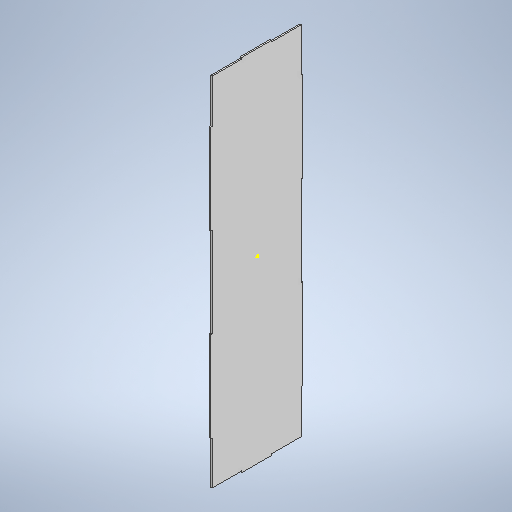
# Autodesk Inventor part: PAREDES LATERAIS
Saved by Autodesk Inventor 2025.2 (Build 292293000, 293)
## iProperties
Created: 2025-05-08
Part Number: PAREDES LATERAIS
Material: Genérico
Document SubType Name: Modeling
Designer: erick
Density: 1 g/cm^3
Appearance: Padrão
Author: erick
Autodesk Inventor part; units mm, degrees
ref_plane "YZ Plane" through (0, 0, 0) normal (1, 0, 0) x (0, 1, 0)
ref_plane "XZ Plane" through (0, 0, 0) normal (0, 1, 0) x (-1, 0, 0)
ref_plane "XY Plane" through (0, 0, 0) normal (0, 0, 1) x (1, 0, 0)
sketch "Esboço1" plane through (0, 0, 0) normal (1, 0, 0) x (0, 1, 0)
  line L0 (-504, 129) -> (504, 129)
  line L1 (504, 129) -> (504, -129)
  line L2 (504, -129) -> (-504, -129)
  line L3 (-504, -129) -> (-504, 129)
  line L4 (-504, 129) -> (504, -129) construction
  line L5 (504, 129) -> (-504, -129) construction
  point P0 (0, 0)
  dimension "d0" = 1008
  dimension "d1" = 258
  constraints: 12 end point, 2 midpoint, 2 parallel, 1 horizontal, 1 perpendicular
  measures "d0" distance of L1.end L2.end
  measures "d1" distance of L0.end L1.end
extrude "Extrusão1" add sketch "Esboço1" along normal mid plane 4
sketch "Esboço3" plane through (2, 0, 0) normal (1, 0, 0) x (0, 0, -1)
  line L0 (-133, 630) -> (-125, 630)
  line L1 (-125, 630) -> (-125, 378)
  line L2 (-125, 378) -> (-133, 378)
  line L3 (-133, 378) -> (-133, 630)
  line L4 (129, 504) -> (-129, 504) projected
  line L5 (-133, 630) -> (-125, 378) construction
  line L6 (-125, 630) -> (-133, 378) construction
  line L7 (-125, 126) -> (-133, 126)
  line L8 (-133, 126) -> (-133, -126)
  line L9 (-133, -126) -> (-125, -126)
  line L10 (-125, -126) -> (-125, 126)
  line L11 (-129, 504) -> (-129, -504) projected
  line L12 (-125, 126) -> (-133, -126) construction
  line L13 (-133, 126) -> (-125, -126) construction
  line L14 (-125, -378) -> (-133, -378)
  line L15 (-133, -378) -> (-133, -630)
  line L16 (-133, -630) -> (-125, -630)
  line L17 (-125, -630) -> (-125, -378)
  line L18 (-125, -378) -> (-133, -630) construction
  line L19 (-133, -378) -> (-125, -630) construction
  line L20 (125, 630) -> (133, 630)
  line L21 (133, 630) -> (133, 378)
  line L22 (133, 378) -> (125, 378)
  line L23 (125, 378) -> (125, 630)
  line L24 (125, 630) -> (133, 378) construction
  line L25 (133, 630) -> (125, 378) construction
  line L26 (125, 126) -> (133, 126)
  line L27 (133, 126) -> (133, -126)
  line L28 (133, -126) -> (125, -126)
  line L29 (125, -126) -> (125, 126)
  line L30 (129, -504) -> (129, 504) projected
  line L31 (125, 126) -> (133, -126) construction
  line L32 (133, 126) -> (125, -126) construction
  line L33 (125, -378) -> (133, -378)
  line L34 (133, -378) -> (133, -630)
  line L35 (133, -630) -> (125, -630)
  line L36 (125, -630) -> (125, -378)
  line L37 (125, -378) -> (133, -630) construction
  line L38 (133, -378) -> (125, -630) construction
  point P0 (0, 0)
  point P1 (-129, 0)
  point P2 (-129, -504)
  point P3 (129, 0)
  dimension "d8" = 8
  dimension "d9" = 252
  dimension "d10" = 252
  dimension "d11" = 252
  dimension "d12" = 8
  dimension "d13" = 252
  dimension "d14" = 8
  dimension "d15" = 252
  dimension "d16" = 8
  dimension "d17" = 252
  dimension "d18" = 252
  dimension "d19" = 8
  dimension "d20" = 252
  dimension "d21" = 252
  dimension "d22" = 8
  dimension "d23" = 252
  constraints: 72 end point, 14 midpoint, 12 parallel, 6 horizontal, 6 perpendicular, 1 point on line
  measures "d8" distance of L0.start L0.end
  measures "d9" distance of L0.end L1.end
  measures "d10" distance of L9.end L7.start
  measures "d11" distance between parallel lines of L7 L2
  measures "d12" distance of L8.end L9.end
  measures "d13" distance between parallel lines of L14 L9
  measures "d14" distance of L14.start L14.end
  measures "d15" distance of L16.end L14.start
  measures "d16" distance of L21.end L22.end
  measures "d17" distance of L20.end L21.end
  measures "d18" distance between parallel lines of L26 L22
  measures "d19" distance of L26.start L26.end
  measures "d20" distance of L26.end L27.end
  measures "d21" distance of L33.end L34.end
  measures "d22" distance of L33.start L33.end
  measures "d23" distance between parallel lines of L33 L28
extrude "Extrusão3" cut sketch "Esboço3" along normal through all both and the other way through all
sketch "Esboço4" plane through (2, 0, 0) normal (1, 0, 0) x (0, 0, -1)
  line L0 (-125, 504) -> (125, 504) projected
  line L1 (-125, 504) -> (-42, 504)
  line L2 (-42, 504) -> (-42, 500)
  line L3 (-42, 500) -> (-125, 500)
  line L4 (-125, 500) -> (-125, 504)
  line L5 (125, 504) -> (42, 504)
  line L6 (42, 504) -> (42, 500)
  line L7 (42, 500) -> (125, 500)
  line L8 (125, 500) -> (125, 504)
  line L9 (-125, -504) -> (125, -504) projected
  line L10 (-125, -504) -> (-42, -504)
  line L11 (-42, -504) -> (-42, -500)
  line L12 (-42, -500) -> (-125, -500)
  line L13 (-125, -500) -> (-125, -504)
  line L14 (125, -504) -> (42, -504)
  line L15 (42, -504) -> (42, -500)
  line L16 (42, -500) -> (125, -500)
  line L17 (125, -500) -> (125, -504)
  point P0 (0, 0)
  dimension "d26" = 83
  dimension "d27" = 4
  dimension "d28" = 83
  dimension "d29" = 4
  dimension "d30" = 84
  dimension "d31" = 83
  dimension "d32" = 4
  dimension "d33" = 83
  dimension "d34" = 4
  dimension "d35" = 84
  constraints: 32 end point, 8 parallel, 4 horizontal, 4 perpendicular
  measures "d26" distance of L2.end L3.end
  measures "d27" distance of L1.end L2.end
  measures "d28" distance of L6.end L7.end
  measures "d29" distance of L5.end L6.end
  measures "d30" distance between parallel lines of L6 L2
  measures "d31" distance of L11.end L12.end
  measures "d32" distance of L10.end L11.end
  measures "d33" distance of L15.end L16.end
  measures "d34" distance of L14.end L15.end
  measures "d35" distance between parallel lines of L15 L11
extrude "Extrusão4" cut sketch "Esboço4" along normal through all both and the other way through all
sketch "Esboço6" plane through (2, 0, 0) normal (1, 0, 0) x (0, 0, -1)
  point P0 (0, 0)
